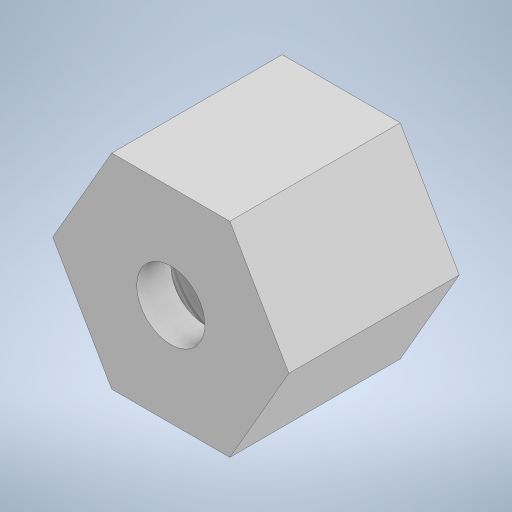
# Autodesk Inventor part: HUDSON-1-80
Saved by Autodesk Inventor 2024.2 (Build 282272000, 272)
## iProperties
Created: 2024-10-06
Part Number: HUDSON-1-80
Material: Generic
Document SubType Name: Modeling
Designer: melim
Density: 1 g/cm^3
Appearance: Default
Author: melim
Autodesk Inventor part; units mm, degrees
ref_plane "YZ Plane" through (0, 0, 0) normal (1, 0, 0) x (0, 1, 0)
ref_plane "XZ Plane" through (0, 0, 0) normal (0, 1, 0) x (-1, 0, 0)
ref_plane "XY Plane" through (0, 0, 0) normal (0, 0, 1) x (1, 0, 0)
sketch "Sketch1" plane through (0, 0, 0) normal (0, 0, 1) x (1, 0, 0)
  line L0 (0, 0) -> (0, -17) construction
  line L1 (-3.4641, -6) -> (-6.9282, 0)
  line L2 (-6.9282, 0) -> (-3.4641, 6)
  line L3 (-3.4641, 6) -> (3.4641, 6)
  line L4 (3.4641, 6) -> (6.9282, 0)
  line L5 (6.9282, 0) -> (3.4641, -6)
  line L6 (3.4641, -6) -> (-3.4641, -6)
  point P0 (0, -6)
  dimension "d0" = 12
  constraints: 14 end point, 1 coincident, 1 midpoint, 1 point on line, 1 vertical, 13 other
  measures "d0" distance between parallel lines of L5 L2
extrude "Extrusion1" add sketch "Sketch1" along normal blind 10
hole "Hole1" at (0, 0, 0) direction (0, 0, 1) diameter 4 end through all counterbore diameter 8 counterbore depth 8
thread "Thread1" size "M8x1.25" class "6H" standard "ANSI Metric M Profile" full length
body "Solid1"
